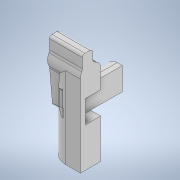
# Autodesk Inventor part: ДИ 00.00.02
Saved by Autodesk Inventor 2021.2 (Build 252289000, 289)
## iProperties
Created: 2021-10-11
Part Number: ДИ 00.00.02
Material: Типовые
Document SubType Name: Modeling
Designer: Surflay
Density: 1 g/cm^3
Appearance: По умолчанию
Author: Surflay
Autodesk Inventor part; units mm, degrees
ref_plane "YZ Plane" through (0, 0, 0) normal (1, 0, 0) x (0, 1, 0)
ref_plane "XZ Plane" through (0, 0, 0) normal (0, 1, 0) x (-1, 0, 0)
ref_plane "XY Plane" through (0, 0, 0) normal (0, 0, 1) x (1, 0, 0)
sketch "Эскиз1" plane through (0, 0, 0) normal (0, 0, 1) x (1, 0, 0)
  line L0 (0, 0) -> (-30, 0)
  line L1 (-30, 0) -> (-30, -45)
  line L2 (-30, -45) -> (0, -45)
  line L3 (0, -45) -> (0, 0)
  dimension "d0" = 30
  dimension "d1" = 45
  constraints: 8 end point, 2 parallel, 1 horizontal, 1 perpendicular
  measures "d0" distance of L2.end L1.end
  measures "d1" distance of L1.end L0.end
extrude "Выдавливание1" add sketch "Эскиз1" along normal blind 38
sketch "Эскиз2" plane through (0, 0, 38) normal (0, 0, 1) x (1, 0, 0)
  line L0 (0, -45) -> (0, 0) projected
  line L1 (-30, -45) -> (0, -45) projected
  line L2 (0, 0) -> (-44, 0)
  line L3 (-44, 0) -> (-44, -45)
  line L4 (-44, -45) -> (0, -45)
  line L5 (0, -45) -> (0, 0)
  dimension "d4" = 44
  constraints: 8 end point, 2 parallel, 1 horizontal, 1 perpendicular, 1 point on line
  measures "d4" distance of L4.end L3.end
extrude "Выдавливание2" add sketch "Эскиз2" along normal blind 65
sketch "Эскиз3" plane through (0, -45, 0) normal (1, 0, 0) x (0, 0, -1)
  line L0 (0, 0) -> (-103, 0) projected
  line L1 (0, 45) -> (-103, 45) projected
  line L2 (-103, 0) -> (-93, 0)
  line L3 (-93, 0) -> (-93, 45)
  line L4 (-93, 45) -> (-103, 45)
  line L5 (-103, 45) -> (-103, 0)
  dimension "d7" = 10
  constraints: 8 end point, 2 parallel, 1 horizontal, 1 perpendicular, 1 point on line
  measures "d7" distance of L4.end L3.end
extrude "Выдавливание3" add sketch "Эскиз3" along normal blind 90
sketch "Эскиз5" plane through (-30, -45, 0) normal (0, -1, 0) x (1, 0, 0)
  line L0 (-14, 103) -> (120, 103)
  line L1 (120, 103) -> (120, 63)
  line L2 (120, 63) -> (-14, 63)
  line L3 (-14, 63) -> (-14, 103)
  line L4 (-14, 38) -> (-14, 103) projected
  point P0 (30, 0)
  point P1 (16, 50.0711)
  point P2 (-4, 93)
  point P3 (1, 38)
  dimension "d18" = 40
  constraints: 8 end point, 2 parallel, 1 coincident, 1 horizontal, 1 perpendicular, 2 other
  measures "d18" distance of L0.end L1.end
extrude "Выдавливание5" add sketch "Эскиз5" along normal blind 78
sketch "Эскиз6" plane through (-30, 0, 0) normal (0, 1, 0) x (1, 0, 0)
  line L0 (30, -63) -> (120, -63) projected
  line L1 (-14, -103) -> (120, -103)
  line L2 (120, -103) -> (120, -63)
  line L3 (120, -63) -> (-14, -63)
  line L4 (-14, -63) -> (-14, -103)
  point P0 (30, 0)
  point P1 (1, -63)
  constraints: 8 end point, 2 parallel, 1 horizontal, 1 perpendicular
extrude "Выдавливание6" add sketch "Эскиз6" along normal blind 78
sketch "Эскиз7" plane through (-44, -45, 38) normal (-1, 0, 0) x (0, 0, 1)
  line L0 (65, -78) -> (65, 123) projected
  line L1 (65, 123) -> (25, 123) projected
  line L2 (61.0947, 118) -> (61.0947, 99)
  line L3 (55, 0) -> (55, 45) projected
  line L4 (60.8993, 67.4298) -> (55.4358, 4.981)
  line L5 (50.019, 0.4358) -> (29.1318, 2.2632)
  line L6 (25, 45) -> (25, 123) projected
  line L7 (25, 59.0042) -> (25, 83)
  line L8 (41.0947, 106.5465) -> (41.0947, 118)
  line L9 (56.0947, 123) -> (46.0947, 123)
  line L10 (25, 0) -> (55, 0) projected
  arc A0 (50.019, 0.4358) -> (55.4358, 4.981) centre (50.4548, 5.4168) ccw
  line L11 (29.1318, 2.2632) -> (4.1318, 6.6714)
  line L12 (0, 45) -> (0, 0) projected
  line L13 (0, 11.5954) -> (0, 32.3997)
  line L14 (3.2899, 37.0982) -> (11.8404, 40.2103)
  arc A1 (11.8404, 40.2103) -> (25, 59.0042) centre (5, 59.0042) ccw
  line L15 (0, 0) -> (25, 0) projected
  line L16 (0, 45) -> (25, 45) projected
  arc A2 (3.2899, 37.0982) -> (0, 32.3997) centre (5, 32.3997) ccw
  arc A3 (0, 11.5954) -> (4.1318, 6.6714) centre (5, 11.5954) ccw
  arc A4 (62.053, 71.2926) -> (62.2192, 94.3928) centre (40.2717, 83) ccw
  arc A5 (34.726, 97.2292) -> (25, 83) centre (40.2717, 83) ccw
  arc A6 (61.0947, 99) -> (62.2192, 94.3928) centre (71.0947, 99) ccw
  arc A7 (62.053, 71.2926) -> (60.8993, 67.4298) centre (70.8613, 66.5582) ccw
  arc A8 (34.726, 97.2292) -> (41.0947, 106.5465) centre (31.0947, 106.5465) ccw
  arc A9 (46.0947, 123) -> (41.0947, 118) centre (46.0947, 118) ccw
  arc A10 (61.0947, 118) -> (56.0947, 123) centre (56.0947, 118) ccw
  point P0 (-38, 45)
  point P1 (61.0947, 123)
  point P2 (61.0947, 96.3377)
  point P3 (61.0947, 69.6623)
  point P4 (41.0947, 98.2495)
  point P5 (41.0947, 123)
  point P6 (0, 7.3999)
  point P7 (46.0947, 123)
  point P8 (19.2788, 45)
  dimension "d23" = 5
  dimension "d24" = 5
  dimension "d25" = 40
  dimension "d27" = 20
  dimension "d29" = 5
  dimension "d30" = 20
  dimension "d31" = 10
  dimension "d32" = 20
  dimension "d33" = 5
  dimension "d34" = 25
  dimension "d35" = 10
  dimension "d36" = 5
  dimension "d37" = 19
  constraints: 25 point on circle, 20 tangent, 18 end point, 18 point on line, 11 centre point, 4 equal radius, 2 perpendicular, 1 collinear, 1 vertical
  measures "d23" angle of L10 L5
  measures "d24" angle of L0 L4
  measures "d25" distance from line of A4.centre L1
  measures "d27" distance between parallel lines of L8 L2
  measures "d29" radius of A0
  measures "d30" radius of A1
  measures "d31" angle of L15 L11
  measures "d32" angle of L16 L14
  measures "d33" radius of A2
  measures "d34" horizontal distance of L5.end L11.end
  measures "d35" radius of A6
  measures "d36" radius of A9
  measures "d37" distance of L2.start L2.end
extrude "Выдавливание7" add sketch "Эскиз7" along normal blind 1 contours A4 A7 L4 A0 L5 L11 A3 L12 A2 L14 A1 L16 L6 A5 A8 L8 A9 L1 A10 L2 A6
sketch "Эскиз8" plane through (-44, -12.6003, 38) normal (-1, 0, 0) x (0, 0, 1)
  arc A0 (11.8404, 7.8106) -> (19.2788, 12.6003) centre (5, 26.6044) ccw projected
  line L0 (11.8404, 7.8106) -> (3.2899, 4.6985) projected
  arc A1 (3.2899, 4.6985) -> (0, 0) centre (5, 0) ccw projected
  line L1 (0, 12.6003) -> (0, 0) projected
  arc A2 (3.2899, 4.6985) -> (0, 0) centre (5, 0) ccw projected
  line L2 (3.2899, 4.6985) -> (11.8404, 7.8106) projected
  arc A3 (11.8404, 7.8106) -> (19.2788, 12.6003) centre (5, 26.6044) ccw projected
  line L3 (0, 12.6003) -> (19.2788, 12.6003) projected
  line L4 (0, 12.6003) -> (0, 0) projected
  point P0 (-38, 12.6003)
  point P1 (19.2788, 12.6003)
extrude "Выдавливание8" cut sketch "Эскиз8" against normal up to surface (14 mm away)
sketch "Эскиз9" plane through (-44, -123, 63) normal (-1, 0, 0) x (0, 0, 1)
  line L0 (25.019, 78.4358) -> (4.1318, 80.2632) projected
  line L1 (4.1318, 80.2632) -> (-20.8682, 84.6714) projected
  arc A0 (-25, 89.5954) -> (-20.8682, 84.6714) centre (-20, 89.5954) ccw projected
  line L2 (-25, 89.5954) -> (-25, 78) projected
  line L3 (-25, 78) -> (0, 78) projected
  line L4 (0, 78) -> (0, 0) projected
  line L5 (40, 0) -> (0, 0) projected
  line L6 (-20.8682, 84.6714) -> (4.1318, 80.2632) projected
  line L7 (0, 80.9917) -> (0, 78)
  line L8 (40, 0) -> (40, 161) projected
  arc A1 (37.053, 149.2926) -> (40, 161) centre (15.2717, 161) ccw projected
  arc A2 (37.053, 149.2926) -> (35.8993, 145.4298) centre (45.8613, 144.5582) ccw projected
  line L9 (35.8993, 145.4298) -> (30.4358, 82.981) projected
  arc A3 (25.019, 78.4358) -> (30.4358, 82.981) centre (25.4548, 83.4168) ccw projected
  point P0 (-63, 123)
  constraints: 2 end point, 1 point on line, 1 vertical
extrude "Выдавливание9" cut sketch "Эскиз9" against normal up to surface (14 mm away) contours L7 L3 L2 A0 L1
sketch "Эскиз10" plane through (-44, 38, 63) normal (-1, 0, 0) x (0, 0, 1)
  arc A0 (9.726, 14.2292) -> (0, 0) centre (15.2717, 0) ccw projected
  arc A1 (9.726, 14.2292) -> (16.0947, 23.5465) centre (6.0947, 23.5465) ccw projected
  line L0 (16.0947, 23.5465) -> (16.0947, 35) projected
  arc A2 (21.0947, 40) -> (16.0947, 35) centre (21.0947, 35) ccw projected
  line L1 (0, 40) -> (21.0947, 40) projected
  line L2 (0, 0) -> (0, 40) projected
  point P0 (-63, -38)
extrude "Выдавливание10" cut sketch "Эскиз10" against normal through all
sketch "Эскиз11" plane through (-44, 54, 99.0947) normal (-1, 0, 0) x (0, 0, 1)
  line L0 (-0.1953, -31.5702) -> (-5.6589, -94.019) projected
  line L1 (3.9053, -16) -> (3.9053, 24) projected
  line L2 (-5, 24) -> (3.9053, 24) projected
  arc A0 (0, 19) -> (-5, 24) centre (-5, 19) ccw projected
  line L3 (0, 19) -> (0, 0) projected
  arc A1 (0, 0) -> (1.1245, -4.6072) centre (10, 0) ccw projected
  arc A2 (0.9584, -27.7074) -> (3.9053, -16) centre (-20.823, -16) ccw projected
  arc A3 (3.9053, -16) -> (1.1245, -4.6072) centre (-20.823, -16) ccw projected
  line L4 (-36.0947, -96.0083) -> (-36.0947, -177) projected
  line L5 (3.9053, -177) -> (-36.0947, -177) projected
  line L6 (3.9053, -177) -> (3.9053, -16) projected
  arc A4 (0.9584, -27.7074) -> (-0.1953, -31.5702) centre (9.7666, -32.4418) ccw projected
  arc A5 (-11.0756, -98.5642) -> (-5.6589, -94.019) centre (-10.6399, -93.5832) ccw projected
  line L7 (-11.0756, -98.5642) -> (-31.9629, -96.7368) projected
  line L8 (-31.9629, -96.7368) -> (-36.0947, -96.0083) projected
  point P0 (-99.0947, -54)
extrude "Выдавливание11" cut sketch "Эскиз11" against normal through all contours A3 A1 L3 A0 L2 L1
fillet "Сопряжение4" radius 35 1 edges at (-44, -42.5, 103)
ref_plane "РабПлоскость1" through (-25, -45, 38) normal (-1, 0, 0) x (0, 0, 1)
sketch "Эскиз12" plane through (-25, -45, 38) normal (-1, 0, 0) x (0, 0, 1)
  line L0 (65, -78) -> (65, 83) projected
  line L1 (65, 48) -> (64.1272, -2)
  line L2 (60, 41) -> (60, 11)
  line L3 (60, 41) -> (65, 48)
  line L4 (60, 11) -> (64.1272, -2)
  point P0 (-38, 45)
  dimension "d62" = 35
  dimension "d63" = 50
  dimension "d64" = 30
  dimension "d65" = 5
  dimension "d66" = 1
  dimension "d67" = 126.849
  constraints: 8 end point, 1 point on line, 1 vertical
  measures "d62" distance of L0.end L1.start
  measures "d63" vertical distance of L1.start L1.end
  measures "d64" distance of L2.start L2.end
  measures "d65" horizontal distance of L1.start L2.start
  measures "d66" angle of L0 L1
  measures "d67" angle of L3 L4
extrude "Выдавливание12" cut sketch "Эскиз12" against normal mid plane 20
fillet "Сопряжение5" radius 20 1 edges at (-30, -45, 31.5)
fillet "Сопряжение6" radius 20 1 edges at (-30, 0, 28.6394)
sketch "Эскиз13" plane through (0, 0, 103) normal (0, 0, 1) x (1, 0, 0)
  line L0 (90, 78) -> (-45, 78) projected
  line L1 (90, -45) -> (90, -123) projected
  line L2 (20, 78) -> (90, 78)
  line L3 (90, 78) -> (90, -123)
  line L4 (90, -123) -> (20, -123)
  line L5 (20, -123) -> (20, 78)
  point P0 (0, 0)
  dimension "d70" = 70
  constraints: 8 end point, 2 parallel, 1 horizontal, 1 perpendicular, 1 point on line
  measures "d70" distance between parallel lines of L3 L5
extrude "Выдавливание13" cut sketch "Эскиз13" against normal through all
